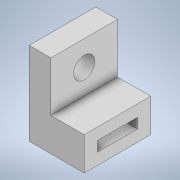
# Autodesk Inventor part: adjustment_2-6
Saved by Autodesk Inventor 2020 (Build 240168000, 168)
## iProperties
Created: 2020-02-07
Part Number: adjustment_2-6
Material: Generic
Document SubType Name: Modeling
Designer: akend
Density: 1 g/cm^3
Appearance: Default
Author: akend
## iProperties of the stored document _3DPrint.ipt
Created: 2020-02-07
Part Number: _3DPrint
Material: Generic
Document SubType Name: Modeling
Designer: akend
Density: 1 g/cm^3
Appearance: Default
Author: akend
Autodesk Inventor part; units mm, degrees
ref_plane "YZ Plane" through (0, 0, 0) normal (1, 0, 0) x (0, 1, 0)
ref_plane "XZ Plane" through (0, 0, 0) normal (0, 1, 0) x (-1, 0, 0)
ref_plane "XY Plane" through (0, 0, 0) normal (0, 0, 1) x (1, 0, 0)
sketch "Sketch1" plane through (0, 0, 0) normal (1, 0, 0) x (0, 1, 0)
  line L0 (0, 0) -> (25, 0)
  line L1 (25, 0) -> (25, -20)
  line L2 (25, -20) -> (0, -20)
  line L3 (0, -20) -> (0, 0)
  line L4 (3.5, -4) -> (6.5, -4)
  line L5 (6.5, -4) -> (6.5, -16)
  line L6 (6.5, -16) -> (3.5, -16)
  line L7 (3.5, -16) -> (3.5, -4)
  dimension "d0" = 25
  dimension "d1" = 20
  dimension "d2" = 3
  dimension "d3" = 12
  constraints: 16 end point, 4 parallel, 2 horizontal, 2 perpendicular
  measures "d0" distance of L1.end L2.end
  measures "d1" distance of L0.end L1.end
  measures "d2" distance of L5.end L6.end
  measures "d3" distance of L4.end L5.end
extrude "Extrusion1" add sketch "Sketch1" along normal blind 6.5
sketch "Sketch2" plane through (6.5, 0, 0) normal (1, 0, 0) x (0, 0, -1)
  line L0 (0, 25) -> (0, 0) projected
  line L1 (20, 0) -> (20, 25) projected
  line L2 (0, 0) -> (20, 0)
  line L3 (20, 0) -> (20, 10)
  line L4 (20, 10) -> (0, 10)
  line L5 (0, 10) -> (0, 0)
  line L6 (4, 3.5) -> (4, 6.5) projected
  line L7 (4, 6.5) -> (16, 6.5) projected
  line L8 (4, 3.5) -> (16, 3.5)
  line L9 (16, 3.5) -> (16, 6.5)
  line L10 (16, 6.5) -> (4, 6.5)
  line L11 (4, 6.5) -> (4, 3.5)
  dimension "d6" = 10
  constraints: 16 end point, 4 parallel, 2 horizontal, 2 perpendicular, 1 point on line
  measures "d6" distance of L3.end L2.end
extrude "Extrusion2" add sketch "Sketch2" along normal blind 10
sketch "Sketch3" plane through (6.5, 0, 0) normal (1, 0, 0) x (0, 0, -1)
  line L0 (20, 0) -> (20, 25) construction
  line L1 (0, 10) -> (0, 0) construction
  line L2 (20, 25) -> (0, 10) construction
  circle A0 centre (10, 17.5) radius 3.2
  dimension "d9" = 6.4
  constraints: 2 end point, 1 centre point, 1 midpoint
  measures "d9" diameter of A0
extrude "Extrusion3" cut sketch "Sketch3" against normal blind 10
body "Solid1"
